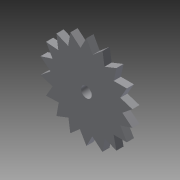
# Autodesk Inventor part: zebatka
Saved by Autodesk Inventor 2014 (Build 180170000, 170)
## iProperties
Created: 2013-10-14
Part Number: zebatka
Material: Stal
Document SubType Name: Modeling
Designer: Wojciech
Density: 7.85 g/cm^3
Appearance: Stal
Mass: 6.26846 g
Surface Area: 10.7655 cm^2
Volume: 0.79853 cm^3
Author: Wojciech
Autodesk Inventor part; units mm, degrees
ref_plane "YZ Plane" through (0, 0, 0) normal (1, 0, 0) x (0, 1, 0)
ref_plane "XZ Plane" through (0, 0, 0) normal (0, 1, 0) x (-1, 0, 0)
ref_plane "XY Plane" through (0, 0, 0) normal (0, 0, 1) x (1, 0, 0)
sketch "Szkic1" plane through (0, 0, 0) normal (0, 1, 0) x (-1, 0, 0)
  line L0 (0, 12.8914) -> (0, 13)
  line L1 (4.409, 12.114) -> (4.4461, 12.216)
  line L2 (0, 0) -> (13, 0) construction
  line L3 (0, 0) -> (13, 0) construction
  line L4 (12.8025, -2.2574) -> (12.7826, -2.312)
  line L5 (0, -13) -> (0.0571, -12.9898)
  line L6 (0, 13) -> (-1.7143, 9.8513)
  line L7 (-4.506, 12.1936) -> (-1.7143, 9.8513)
  line L8 (-4.506, 12.1936) -> (-5.0309, 8.6423)
  line L9 (-5.0309, 8.6423) -> (-8.3572, 9.9584)
  line L10 (-8.3572, 9.9584) -> (-7.5993, 6.5)
  line L11 (-11.2583, 6.5) -> (-7.5993, 6.5)
  line L12 (-12.8025, 2.2574) -> (-9.4249, 3.3421)
  line L13 (-11.2583, 6.5) -> (-9.4249, 3.3421)
  line L14 (-12.8025, 2.2574) -> (-10, -0.0042)
  line L15 (-12.8025, -2.2574) -> (-10, -0.0042)
  line L16 (-4.4461, -12.216) -> (-1.6431, -9.864)
  line L17 (0, -13) -> (-1.6431, -9.864)
  line L18 (4.5054, -12.1944) -> (1.8242, -9.8405)
  line L19 (1.8242, -9.8405) -> (0, -13)
  line L20 (-8.3562, -9.9586) -> (-5.0917, -8.6067)
  line L21 (-4.4461, -12.216) -> (-5.0917, -8.6067)
  line L22 (-8.3562, -9.9586) -> (-7.5993, -6.5)
  line L23 (-11.2583, -6.5) -> (-7.5993, -6.5)
  line L24 (-11.2583, -6.5) -> (-9.4288, -3.3312)
  line L25 (-12.8025, -2.2574) -> (-9.4288, -3.3312)
  line L26 (4.5054, -12.1944) -> (4.9903, -8.6659)
  line L27 (8.3572, -9.9584) -> (4.9903, -8.6659)
  line L28 (8.3572, -9.9584) -> (7.7142, -6.364)
  line L29 (11.2583, -6.5) -> (7.7142, -6.364)
  line L30 (11.2583, -6.5) -> (9.425, -3.3422)
  line L31 (12.8025, -2.2574) -> (9.425, -3.3422)
  line L32 (0, 13) -> (1.6431, 9.864)
  line L33 (1.6431, 9.864) -> (4.4461, 12.216)
  line L34 (4.4461, 12.216) -> (5.0917, 8.6067)
  line L35 (8.3562, 9.9586) -> (5.0917, 8.6067)
  line L36 (8.3562, 9.9586) -> (7.8406, 6.2068)
  line L37 (11.2583, 6.5) -> (7.8406, 6.2068)
  line L38 (12.8025, 2.2574) -> (9.4288, 3.3312)
  line L39 (11.2583, 6.5) -> (9.4288, 3.3312)
  line L40 (12.8025, -2.2574) -> (10, 0)
  line L41 (12.8025, 2.2574) -> (10, 0)
  line L42 (-0.0571, 12.9898) -> (0, 13)
  arc A0 (5.0917, 8.6067) -> (5.0298, 8.643) centre (0, 0) ccw
  line L43 (-8.4028, 9.904) -> (-8.3572, 9.9584)
  line L44 (8.4028, -9.904) -> (8.3572, -9.9584)
  constraints: 90 end point, 15 parallel, 9 point on line, 2 coincident, 2 horizontal, 2 perpendicular, 2 point on circle, 1 centre point, 1 vertical
extrude "Wyciągnięcie proste1" add sketch "Szkic1" along normal blind 2
sketch "Szkic2" plane through (0, 2, 0) normal (0, 1, 0) x (1, 0, 0)
  circle A0 centre (0, 0) radius 1.5
  dimension "d9" = 3
  constraints: 1 centre point, 1 coincident
  measures "d9" diameter of A0
hole "Otwór1" at (0, 2, 0) direction (0, -1, 0) diameter 3 depth 8 tip angle 118
